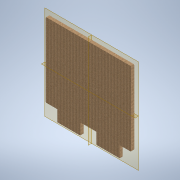
# Autodesk Inventor part: Side_Side_MDF
Saved by Autodesk Inventor 2021 (Build 250183000, 183)
## iProperties
Created: 2021-02-17
Part Number: Side_Side_MDF
Material: MDF Medium Density Fiberboard
Document SubType Name: Modeling
Designer: negt20
Density: 0.8 g/cm^3
Appearance: Cardboard - Corrugated
Author: negt20
Autodesk Inventor part; units mm, degrees
sketch "Sketch1" plane through (0, 0, 0) normal (0, 0, 1) x (1, 0, 0)
  line L0 (-80.5, 80.75) -> (80.5, 80.75)
  line L1 (80.5, 80.75) -> (80.5, -80.75)
  line L2 (80.5, -80.75) -> (-80.5, -80.75)
  line L3 (-80.5, -80.75) -> (-80.5, 80.75)
  point P0 (0, 80.75)
  point P1 (0, 0)
  point P2 (-80.5, 0)
  dimension "d0" = 161
  dimension "d1" = 161.5
  constraints: 8 end point, 2 midpoint, 2 parallel, 1 horizontal, 1 horizontal alignment, 1 perpendicular, 1 vertical alignment
  measures "d0" distance of L1.end L2.end
  measures "d1" distance of L0.end L1.end
extrude "Extrusion1" add sketch "Sketch1" along normal blind 6
sketch "Sketch2" plane through (0, 0, 6) normal (0, 0, 1) x (1, 0, 0)
  line L0 (-80.5, 80.75) -> (-80.5, -80.75) projected
  line L1 (-80.5, -80.75) -> (-80.5, -59.25)
  line L2 (-80.5, -59.25) -> (-59, -59.25)
  line L3 (-80.5, -80.75) -> (80.5, -80.75) projected
  line L4 (-59, -59.25) -> (-59, -80.75)
  line L5 (-80.5, -80.75) -> (-59, -80.75)
  point P0 (0, 0)
  point P1 (40.5, -62.5)
  point P2 (-64.5, -80.75)
  dimension "d14" = 21.5
  dimension "d15" = 21.5
  constraints: 8 end point, 1 horizontal, 1 perpendicular, 1 point on line, 1 vertical, 3 other
  measures "d14" distance of L0.end L1.end
  measures "d15" distance of L1.end L2.end
extrude "Extrusion2" cut sketch "Sketch2" against normal blind 15
mirror "Mirror1" about plane through (0, 0, 0) normal (1, 0, 0) of "Extrusion2"
sketch "Sketch4" plane through (0, 0, 6) normal (0, 0, 1) x (1, 0, 0)
  line L0 (-59, -80.75) -> (59, -80.75) projected
  line L1 (-15, -80.75) -> (15, -80.75)
  line L2 (15, -80.75) -> (15, -59.25)
  line L3 (15, -59.25) -> (-15, -59.25)
  line L4 (-15, -59.25) -> (-15, -80.75)
  point P0 (0, 0)
  point P1 (-64.5, -67.75)
  point P2 (64.5, -67.75)
  point P3 (0, -59.25)
  point P4 (0, -80.75)
  dimension "d18" = 30
  dimension "d19" = 21.5
  constraints: 8 end point, 2 parallel, 1 horizontal, 1 midpoint, 1 perpendicular, 1 vertical alignment, 3 other
  measures "d18" distance of L3.end L2.end
  measures "d19" distance of L2.end L1.end
extrude "Extrusion4" cut sketch "Sketch4" against normal blind 10
fillet "Fillet1" radius 1 8 edges at (-80.5, -59.25, 3) (-15, -80.75, 3) (15, -80.75, 3) (80.5, -59.25, 3) (-15, -59.25, 3) (15, -59.25, 3) (-80.5, 80.75, 3) (80.5, 80.75, 3)
equation "\"d7\" = d5"
equation "\"d5\" = 15"
body "Solid1"
